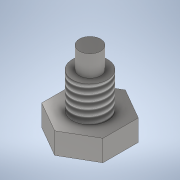
# Autodesk Inventor part: Part20
Saved by Autodesk Inventor 2020 (Build 240168000, 168)
## iProperties
Created: 2021-10-27
Part Number: Part20
Material: Steel, Mild
Document SubType Name: Modeling
Designer: simon.erikssonwestl
Density: 7.85 g/cm^3
Appearance: Semi-Polished
Author: simon.erikssonwestl
Autodesk Inventor part; units mm, degrees
ref_plane "YZ Plane" through (0, 0, 0) normal (1, 0, 0) x (0, 1, 0)
ref_plane "XZ Plane" through (0, 0, 0) normal (0, 1, 0) x (-1, 0, 0)
ref_plane "XY Plane" through (0, 0, 0) normal (0, 0, 1) x (1, 0, 0)
sketch "Sketch1" plane through (0, 0, 0) normal (0, 1, 0) x (-1, 0, 0)
  line L0 (0, -2.5) -> (-2.1651, -1.25)
  line L1 (-2.1651, -1.25) -> (-2.1651, 1.25)
  line L2 (-2.1651, 1.25) -> (0, 2.5)
  line L3 (0, 2.5) -> (2.1651, 1.25)
  line L4 (2.1651, 1.25) -> (2.1651, -1.25)
  line L5 (2.1651, -1.25) -> (0, -2.5)
  point P0 (0, 0)
  point P1 (0, 0)
  dimension "d0" = 5
  constraints: 12 end point, 1 coincident, 13 other
  measures "d0" distance of L2.end L0.start
extrude "Extrusion1" add sketch "Sketch1" along normal blind 1.5
sketch "Sketch2" plane through (0, 1.5, 0) normal (0, 1, 0) x (1, 0, 0)
  circle A0 centre (0, 0) radius 1.25
  dimension "d3" = 2.5
  constraints: 1 centre point, 1 coincident
  measures "d3" diameter of A0
extrude "Extrusion2" add sketch "Sketch2" along normal blind 2.5
thread "Thread1" size "M2.5x0.45" class "6g" standard "ANSI Metric M Profile" length 2.5
sketch "Sketch3" plane through (0, 4, 0) normal (0, 1, 0) x (1, 0, 0)
  circle A0 centre (0, 0) radius 0.75
  dimension "d10" = 1.5
  constraints: 1 centre point, 1 coincident
  measures "d10" diameter of A0
extrude "Extrusion3" add sketch "Sketch3" along normal blind 1.5
body "Solid1"
